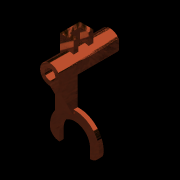
# Autodesk Inventor part: SleevePawl
Saved by Autodesk Inventor 2022 (Build 260153000, 153)
## iProperties
Created: 2020-12-27
Part Number: SleevePawl
Material: Generic
Document SubType Name: Modeling
Designer: jdski
Density: 1 g/cm^3
Appearance: Default
Author: jdski
Autodesk Inventor part; units mm, degrees
ref_plane "YZ Plane" through (0, 0, 0) normal (1, 0, 0) x (0, 1, 0)
ref_plane "XZ Plane" through (0, 0, 0) normal (0, 1, 0) x (-1, 0, 0)
ref_plane "XY Plane" through (0, 0, 0) normal (0, 0, 1) x (1, 0, 0)
sketch "Sketch1" plane through (0, 0, 0) normal (0, 0, 1) x (1, 0, 0)
  arc A0 (9.7668, 0.0221) -> (-9.7912, 0.0221) centre (-0.0122, 0.0221) ccw
  arc A1 (15.7012, -2.2375) -> (-0.806, 15.8772) centre (-0.0122, 0.0221) ccw
  arc A2 (-6.3622, 14.5717) -> (-15.7256, -2.2375) centre (-0.0122, 0.0221) ccw
  line L0 (-0.806, 12.7221) -> (-0.806, 40.4025)
  circle A3 centre (-6.3622, 37.3283) radius 3.429
  arc A4 (-0.806, 40.4025) -> (-0.806, 34.2541) centre (-6.3622, 37.3283) ccw
  line L1 (-12.7122, 37.3283) -> (-12.7122, 9.5471)
  line L2 (-6.3622, 30.9783) -> (-6.3622, 12.7221)
  line L3 (-6.3622, 12.7221) -> (-0.806, 12.7221)
  line L4 (-9.7912, 0.0221) -> (-9.7912, -6.3279)
  line L5 (9.7668, 0.0221) -> (9.7668, -6.3279)
  arc A5 (9.7668, -6.3279) -> (15.7012, -2.2375) centre (9.7668, 0.0221) ccw
  arc A6 (-15.7256, -2.2375) -> (-9.7912, -6.3279) centre (-9.7912, 0.0221) ccw
  line L6 (-12.7122, 37.3283) -> (-12.7122, 50.8221)
  line L7 (-12.7122, 50.8221) -> (-3.981, 50.8221)
  line L8 (-3.981, 50.8221) -> (-3.981, 43.2149)
  constraints: 18 end point, 16 point on circle, 7 centre point, 3 point on line
extrude "Extrusion1" add sketch "Sketch1" along normal blind 9.525 contours L0 L3 L2 A4 | A4 L0
extrude "Extrusion2" add sketch "Sketch1" against normal blind 2.667 contours A0 L4 A6 A2 L2 L3 L0 A1 A5 L5 | L0 L3 L2 A4 | L1 A4 L2 A2
extrude "Extrusion3" add sketch "Sketch1" against normal blind 29.083 contours A4 L0
extrude "Extrusion4" add sketch "Sketch1" against normal blind 15.875 contours L6 L7 L8 A4
extrude "Extrusion5" cut sketch "Sketch1" against normal blind 3.175 contours L6 L7 L8 A4
chamfer "Chamfer1" distance 18.288 distance2 9.3726 1 edges at (-3.5841, 12.7221, 9.525) measured on face at (-3.5841, 13.2221, 9.525)
sketch "Sketch2" plane through (-12.7122, 50.8221, -15.875) normal (0, 1, 0) x (1, 0, 0)
  line L0 (0, 13.208) -> (0, -25.4) projected
  line L1 (8.7313, 0) -> (8.7313, -12.7) projected
  line L2 (0, -12.6995) -> (8.7313, -12.6995)
  line L3 (8.7313, -12.6995) -> (8.7313, 0)
  line L4 (8.7313, 0) -> (0, 0)
  line L5 (0, 0) -> (0, -12.6995)
  line L6 (8.7313, -12.6995) -> (8.7313, -9.6515)
  line L7 (0, 0) -> (0, -12.7) projected
  line L8 (8.7313, -9.6515) -> (3.175, -9.6515)
  line L9 (8.7313, 0) -> (8.7313, -3.048)
  line L10 (8.7313, -3.048) -> (3.175, -3.048)
  line L11 (3.175, -3.048) -> (3.175, -9.6515)
  point P0 (12.7122, -15.875)
  point P1 (8.7313, -3.048)
  dimension "d34" = 3.048
  dimension "d36" = 3.048
  constraints: 18 end point, 4 perpendicular, 3 point on line, 2 parallel, 1 horizontal
  measures "d34" distance of L2.end L6.end
  measures "d36" distance of L1.start L9.end
extrude "Extrusion6" cut sketch "Sketch2" against normal up to surface contours L1 L8 L11 L10 round surface about axis through (-6.3622, 37.3283, 0) along (0, 0, 1) radius 6.35 far side no
body "Solid1"
